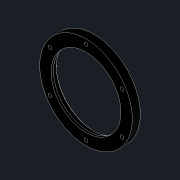
# Autodesk Inventor part: base2
Saved by Autodesk Inventor 2022 (Build 260153000, 153)
## iProperties
Created: 2021-07-17
Part Number: base2
Material: ABS プラスチック
Document SubType Name: Modeling
Designer: yuta0
Density: 1.06 g/cm^3
Appearance: 滑らか - 黒
購入先: 印刷
在庫数: 0.0
Author: yuta0
Autodesk Inventor part; units mm, degrees
ref_plane "YZ Plane" through (0, 0, 0) normal (1, 0, 0) x (0, 1, 0)
ref_plane "XZ Plane" through (0, 0, 0) normal (0, 1, 0) x (-1, 0, 0)
ref_plane "XY Plane" through (0, 0, 0) normal (0, 0, 1) x (1, 0, 0)
sketch "スケッチ1" plane through (0, 0, 0) normal (1, 0, 0) x (0, 1, 0)
  line L0 (32.6, 0) -> (32.6, 5)
  line L1 (32.6, 5) -> (30.6, 5)
  line L2 (30.6, 5) -> (30.6, 7)
  line L3 (30.6, 7) -> (40.6, 7)
  line L4 (40.6, 7) -> (40.6, 0)
  line L5 (40.6, 0) -> (32.6, 0)
  line L6 (0, -1.4) -> (0, 8.4) projected
  point P0 (0, 0)
  dimension "d0" = 32.6
  dimension "d1" = 5
  dimension "d2" = 2
  dimension "d3" = 2
  dimension "d22" = 8
  constraints: 12 end point, 5 perpendicular, 1 horizontal alignment, 1 vertical
  measures "d0" distance from line of point (0, 0) L0
  measures "d1" distance of L0.start L0.end
  measures "d2" distance of L0.end L1.end
  measures "d3" distance of L1.end L2.end
  measures "d22" distance of L4.end L0.start
revolve "回転1" add sketch "スケッチ1" angle 360 about axis through (0, 0, -10) along (0, 0, 1)
sketch "スケッチ2" plane through (0, 0, 7) normal (0, 0, 1) x (1, 0, 0)
  circle A0 centre (0, 0) radius 36.5
  point P0 (0, 36.5)
  point P1 (-31.6099, 18.25)
  point P2 (-31.6099, -18.25)
  point P3 (0, -36.5)
  point P4 (31.6099, -18.25)
  point P5 (31.6099, 18.25)
  dimension "d6" = 73
  dimension "d16" = 360
  constraints: 1 coincident, 1 vertical alignment, 9 other
hole "穴1" at (31.6099, 18.25, 7) at (31.6099, -18.25, 7) at (0, -36.5, 7) at (-31.6099, -18.25, 7) at (-31.6099, 18.25, 7) at (0, 36.5, 7) direction (0, 0, -1) diameter 3.2 end through all clearance for "Socket Head Cap Screw" size "M3" standard "Ansi Metric M Profile"
chamfer "面取り1" distance 0.5 angle 45 1 edges at (0, -32.6, 0)
